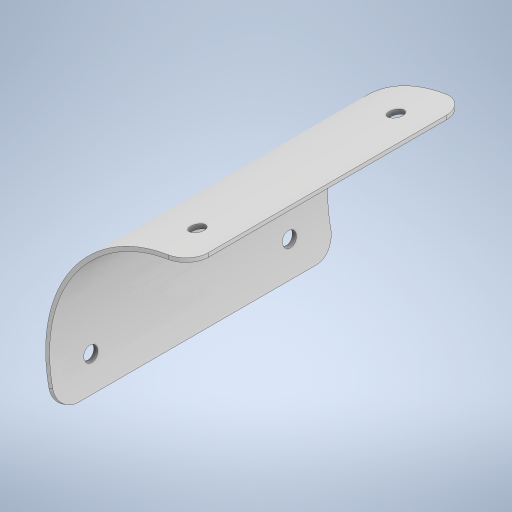
# Autodesk Inventor part: Electronics Door
Saved by Autodesk Inventor 2024 (Build 280153000, 153)
## iProperties
Created: 2024-04-23
Part Number: Electronics Door
Material: Generic
Document SubType Name: Modeling
Designer: auror
Density: 1 g/cm^3
Appearance: Default
Author: auror
Autodesk Inventor part; units mm, degrees
ref_plane "YZ Plane" through (0, 0, 0) normal (1, 0, 0) x (0, 1, 0)
ref_plane "XZ Plane" through (0, 0, 0) normal (0, 1, 0) x (-1, 0, 0)
ref_plane "XY Plane" through (0, 0, 0) normal (0, 0, 1) x (1, 0, 0)
sketch "Sketch1" plane through (0, 0, 0) normal (0, 0, 1) x (1, 0, 0)
  line L0 (0, 39.5237) -> (0, -43.4686) construction
  line L1 (-45.3066, 0) -> (2.8066, 0) construction
  line L2 (-10.604, 34.2765) -> (-34, 0) construction
  line L3 (2.8066, 0) -> (-40.0076, 0) construction
  line L4 (15.8528, -33.3452) -> (-15.0146, 45.5497) construction
  line L5 (2.8066, 0) -> (-40.7672, -15.8596) construction
  arc A0 (-10.2397, 33.3452) -> (-33, 0) centre (2.8066, 0) ccw
  arc A1 (-10.604, 34.2765) -> (-34, 0) centre (2.8066, 0) ccw
  line L6 (1.928, 36.7961) -> (1.928, 35.7958)
  line L7 (-33, 0) -> (-34, 0)
  arc A2 (1.928, 35.7958) -> (-10.2397, 33.3452) centre (2.8066, 0) ccw
  arc A3 (-33, 0) -> (-30.8406, -12.2466) centre (2.8066, 0) ccw
  arc A4 (1.928, 36.7961) -> (-10.604, 34.2765) centre (2.8066, 0) ccw
  arc A5 (-34, 0) -> (-31.7803, -12.5886) centre (2.8066, 0) ccw
  line L8 (-34, 0) -> (-33, 0) construction
  line L9 (-31.7803, -12.5886) -> (-30.8406, -12.2466)
  line L10 (-34, 0) -> (-33, 0)
  line L11 (-10.604, 34.2765) -> (-10.2397, 33.3452)
  line L12 (2.8066, 0) -> (1.608, 50.198) construction
  point P0 (0, 0)
  point P1 (0, 35.5701)
  point P2 (-35.7519, 0.9163)
  dimension "d17" = 41.5
  dimension "d18" = 0
  dimension "d19" = 0
  dimension "d22" = 20
  dimension "d26" = 0
  dimension "d27" = 0
  dimension "d28" = 0
  dimension "d29" = 0
  dimension "d73" = 0
  dimension "d74" = 20
  constraints: 26 end point, 14 point on circle, 11 point on line, 6 centre point, 4 coincident, 4 collinear, 3 vertical, 1 horizontal, 1 perpendicular
  measures "d17" distance of L2.start L2.end
  measures "d18" distance from line of L1 L2.end
  measures "d19" distance from line of L2.end L3
  measures "d22" angle of L5 L1
  measures "d26" distance of L2.end L8.start
  measures "d27" distance of L7.start L8.end
  measures "d28" distance of L2.start L11.start
  measures "d29" distance of A0.start L11.end
  measures "d73" distance from line of L6.start L12
  measures "d74" angle of L12 L4
extrude "Extrusion2" add sketch "Sketch1" along normal blind 70 contours L11 A4 L6 A2
extrude "Extrusion3" add sketch "Sketch1" along normal blind 70 fills toward (-27.5522, 20.7218) open curves A1 L7 A0
extrude "Extrusion4" add sketch "Sketch1" along normal blind 70 contours A3 L9 A5 L7
ref_plane "Work Plane2" through (-10.604, 34.2765, 0) normal (-0.3643541, 0.9312605, 0) x (-0.9312605, -0.3643541, 0)
sketch "Sketch3" plane through (-10.604, 34.2765, 0) normal (-0.3643541, 0.9312605, 0) x (-0.9312605, -0.3643541, 0)
  line L0 (36.7961, 0) -> (-12.5886, 0) projected
  line L1 (-0.001, 0) -> (-0.001, 27.4188)
  point P0 (2.6137, 0)
  point P1 (-5.001, 10)
  dimension "d37" = 10
  dimension "d38" = 5
  constraints: 2 end point, 2 vertical, 1 point on line
  measures "d37" distance from line of L0 point (-5.001, 10)
  measures "d38" distance from line of L1 point (-5.001, 10)
hole "Hole1" at (-5.9468, 36.0987, 10) direction (0.3643541, -0.9312605, 0) diameter 2 end through all counterbore diameter 3.5 counterbore depth 10
sketch "Sketch4" plane through (-10.604, 34.2765, 0) normal (-0.3643541, 0.9312605, 0) x (-0.9312605, -0.3643541, 0)
  line L0 (36.7961, 70) -> (-12.5886, 70) projected
  line L1 (-0.0225, 70) -> (-0.0225, 43.6273)
  point P0 (2.6137, 0)
  point P1 (-5.0225, 60)
  dimension "d46" = 10
  dimension "d47" = 5
  constraints: 2 end point, 2 vertical, 1 point on line
  measures "d46" distance from line of L0 point (-5.022, 60)
  measures "d47" distance from line of L1 point (-5.022, 60)
hole "Hole2" at (-5.9268, 36.1065, 60) direction (0.3643541, -0.9312605, 0) diameter 2 end through all counterbore diameter 3.5 counterbore depth 10
ref_plane "Work Plane3" through (-34, 0, 0) normal (-1, 0, 0) x (0, -1, 0)
sketch "Sketch5" plane through (-34, 0, 0) normal (-1, 0, 0) x (0, -1, 0)
  line L0 (12.5886, 0) -> (-36.7961, 0) projected
  line L1 (0, 0) -> (0, 12.4269)
  point P0 (5, 10)
  dimension "d55" = 10
  dimension "d56" = 5
  constraints: 2 end point, 2 vertical
  measures "d55" distance from line of L0 point (5, 10)
  measures "d56" distance from line of L1 point (5, 10)
hole "Hole3" at (-34, -5, 10) direction (1, 0, 0) diameter 2 end through all counterbore diameter 3.5 counterbore depth 10
sketch "Sketch6" plane through (-34, 0, 0) normal (-1, 0, 0) x (0, -1, 0)
  line L0 (12.5886, 70) -> (-36.7961, 70) projected
  line L1 (0, 70) -> (0, 35.011)
  point P0 (0, 0)
  point P1 (5, 60)
  dimension "d64" = 5
  dimension "d65" = 10
  constraints: 2 end point, 2 vertical, 1 point on line
  measures "d64" distance from line of L1 point (5, 60)
  measures "d65" distance from line of L0 point (5, 60)
hole "Hole4" at (-34, -5, 60) direction (1, 0, 0) diameter 2 end through all counterbore diameter 3.5 counterbore depth 10
fillet "Fillet1" radius 5 1 edges at (1.928, 36.2959, 70)
fillet "Fillet2" radius 5 1 edges at (-31.3104, -12.4176, 70)
fillet "Fillet3" radius 5 1 edges at (1.928, 36.2959, 0)
fillet "Fillet4" radius 5 1 edges at (-31.3104, -12.4176, 0)
body "Solid1"
